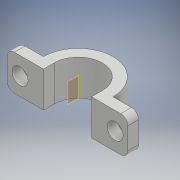
# Autodesk Inventor part: Eletronica - Trava cabo
Saved by Autodesk Inventor 2017 (Build 210142000, 142)
## iProperties
Created: 2020-10-06
Part Number: Eletronica - Trava cabo
Material: Generic
Document SubType Name: Modeling
Designer: ale
Density: 1 g/cm^3
Appearance: Default
Author: ale
Autodesk Inventor part; units mm, degrees
ref_plane "YZ Plane" through (0, 0, 0) normal (1, 0, 0) x (0, 1, 0)
ref_plane "XZ Plane" through (0, 0, 0) normal (0, 1, 0) x (-1, 0, 0)
ref_plane "XY Plane" through (0, 0, 0) normal (0, 0, 1) x (1, 0, 0)
sketch "Sketch1" plane through (0, 0, 0) normal (0, 0, 1) x (1, 0, 0)
  arc A0 (6.75, 0) -> (-6.75, 0) centre (0, 0) ccw
  arc A1 (9.75, 0) -> (-9.75, 0) centre (0, 0) ccw
  line L0 (-6.75, 0) -> (-9.75, 0)
  line L1 (6.75, 0) -> (9.75, 0)
  dimension "d0" = 13.5
  dimension "d1" = 3
  constraints: 4 end point, 4 point on circle, 2 centre point, 2 point on line, 1 coincident, 1 horizontal
  measures "d0" diameter of A0
  measures "d1" radial gap between concentric circles of A0 A1
extrude "Extrusion1" add sketch "Sketch1" along normal blind 10
sketch "Sketch2" plane through (-9.75, 0, 0) normal (0, -1, 0) x (1, 0, 0)
  line L0 (3, 0) -> (3, 10) projected
  line L1 (3, 0) -> (-7.1864, 0)
  line L2 (-7.1864, 0) -> (-7.1864, 10)
  line L3 (-7.1864, 10) -> (3, 10)
  line L4 (3, 10) -> (3, 0)
  point P0 (9.75, 0)
  dimension "d14" = 10
  constraints: 8 end point, 2 parallel, 1 horizontal, 1 perpendicular
  measures "d14" distance between parallel lines of L3 L1
extrude "Extrusion2" add sketch "Sketch2" along normal blind 3
ref_plane "Work Plane1" through (0, -3, 10) normal (1, 0, 0) x (0, 0, -1)
mirror "Mirror1" about plane through (0, -3, 10) normal (1, 0, 0) of "Extrusion2"
sketch "Sketch3" plane through (-9.75, 0, 0) normal (0, 1, 0) x (1, 0, 0)
  line L0 (0, -10) -> (19.5, -10) projected
  line L1 (-7.1864, 0) -> (3, 0) projected
  line L2 (9.75, 0) -> (9.75, -10)
  line L3 (3, -10) -> (16.5, -10) projected
  point P0 (-3.5932, -5)
  point P1 (23.0932, -5)
  dimension "d15" = 5
  constraints: 2 end point, 1 midpoint, 1 symmetric about line
  measures "d15" distance from line of L1 point (-3.593, -5)
hole "Hole1" at (-13.3432, 0, 5) at (13.3432, 0, 5) direction (0, -1, 0) diameter 4.5 end through all
fillet "Fillet1" radius 2 4 edges at (16.9364, -1.5, 10) (16.9364, -1.5, 0) (-16.9364, -1.5, 10) (-16.9364, -1.5, 0)
body "Solid1"
